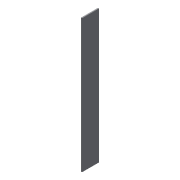
# Autodesk Inventor part: gyro
Saved by Autodesk Inventor 2015 (Build 190159000, 159)
## iProperties
Created: 2015-03-13
Part Number: gyro
Material: Generic
Document SubType Name: Modeling
Designer: Jaden
Density: 1 g/cm^3
Appearance: Default
Author: Jaden
Autodesk Inventor part; units mm, degrees
ref_plane "YZ Plane" through (0, 0, 0) normal (1, 0, 0) x (0, 1, 0)
ref_plane "XZ Plane" through (0, 0, 0) normal (0, 1, 0) x (-1, 0, 0)
ref_plane "XY Plane" through (0, 0, 0) normal (0, 0, 1) x (1, 0, 0)
sketch "Sketch1" plane through (0, 0, 0) normal (0, 0, 1) x (1, 0, 0)
  line L0 (0, 0) -> (0, 396.875)
  line L1 (0, 0) -> (396.875, 0) construction
  line L2 (0, 396.875) -> (3.175, 396.875)
  line L3 (3.175, 396.875) -> (3.175, 0)
  line L4 (3.175, 0) -> (0, 0)
  dimension "d0" = 396.875
  dimension "d1" = 90
  dimension "d2" = 3.175
  constraints: 10 end point, 3 perpendicular, 1 horizontal, 1 parallel, 1 vertical
  measures "d0" distance of L0.start L0.end
  measures "d1" angle of L1 L0
  measures "d2" distance of L0.end L2.end
extrude "Extrusion1" add sketch "Sketch1" along normal blind 50.8
body "Solid1"
